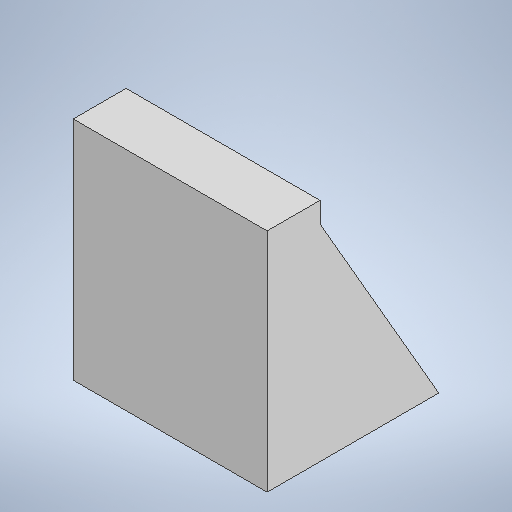
# Autodesk Inventor part: Side near railing 1
Saved by Autodesk Inventor 2025 (Build 290162000, 162)
## iProperties
Created: 2024-07-15
Part Number: Side near railing 1
Material: Generic
Document SubType Name: Modeling
Designer: track
Density: 1 g/cm^3
Appearance: Default
Author: track
Autodesk Inventor part; units mm, degrees
ref_plane "YZ Plane" through (0, 0, 0) normal (1, 0, 0) x (0, 1, 0)
ref_plane "XZ Plane" through (0, 0, 0) normal (0, 1, 0) x (-1, 0, 0)
ref_plane "XY Plane" through (0, 0, 0) normal (0, 0, 1) x (1, 0, 0)
sketch "Sketch1" plane through (0, 0, 0) normal (0, 1, 0) x (-1, 0, 0)
  line L0 (-838.2, 228.6) -> (838.2, 228.6)
  line L1 (838.2, 228.6) -> (838.2, -228.6)
  line L2 (838.2, -228.6) -> (-838.2, -228.6)
  line L3 (-838.2, -228.6) -> (-838.2, 228.6)
  line L4 (-838.2, 228.6) -> (838.2, -228.6) construction
  line L5 (838.2, 228.6) -> (-838.2, -228.6) construction
  point P0 (0, 0)
  dimension "d0" = 1676.4
  dimension "d1" = 457.2
  constraints: 12 end point, 2 midpoint, 2 parallel, 1 horizontal, 1 perpendicular
  measures "d0" distance of L1.end L2.end
  measures "d1" distance of L2.end L0.start
extrude "Extrusion1" add sketch "Sketch1" against normal blind 1955.8
sketch "Sketch2" plane through (838.2, 0, 228.6) normal (1, 0, 0) x (0, 0, -1)
  line L0 (457.2, -177.8) -> (1483.7288, -1955.8)
  line L1 (457.2, -1955.8) -> (0, -1955.8) projected
  line L2 (1483.7288, -1955.8) -> (457.2, -1955.8)
  line L3 (457.2, -1955.8) -> (457.2, -177.8)
  line L4 (0, 0) -> (457.2, 0) projected
  line L5 (457.2, 0) -> (457.2, -1955.8) projected
  point P0 (228.6, 0)
  dimension "d4" = 177.8
  dimension "d5" = 30
  dimension "d6" = 0
  constraints: 6 end point, 1 collinear, 1 perpendicular, 1 point on line
  measures "d4" distance from line of L4 L0.start
  measures "d5" angle of L3 L0
  measures "d6" distance from line of L5 L0.start
extrude "Extrusion2" add sketch "Sketch2" against normal up to surface (1676.4 mm away)
body "Solid1"
